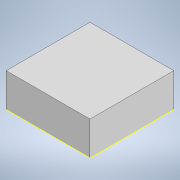
# Autodesk Inventor part: snapfit_lid_v02
Saved by Autodesk Inventor 2022 (Build 260153000, 153)
## iProperties
Created: 2022-03-20
Part Number: snapfit_lid_v02
Material: Generic
Document SubType Name: Modeling
Designer: LIMlab
Density: 1 g/cm^3
Appearance: Default
Author: LIMlab
Autodesk Inventor part; units mm, degrees
ref_plane "YZ Plane" through (0, 0, 0) normal (1, 0, 0) x (0, 1, 0)
ref_plane "XZ Plane" through (0, 0, 0) normal (0, 1, 0) x (-1, 0, 0)
ref_plane "XY Plane" through (0, 0, 0) normal (0, 0, 1) x (1, 0, 0)
sketch "Sketch1" plane through (0, 0, 0) normal (0, 1, 0) x (-1, 0, 0)
  line L0 (-2.5, 2.5) -> (2.5, 2.5)
  line L1 (2.5, 2.5) -> (2.5, -2.5)
  line L2 (2.5, -2.5) -> (-2.5, -2.5)
  line L3 (-2.5, -2.5) -> (-2.5, 2.5)
  line L4 (-2.5, 2.5) -> (2.5, -2.5) construction
  line L5 (2.5, 2.5) -> (-2.5, -2.5) construction
  point P0 (0, 0)
  dimension "d0" = 5
  dimension "d1" = 5
  constraints: 12 end point, 2 midpoint, 2 parallel, 1 horizontal, 1 perpendicular
  measures "d0" distance of L0.end L1.end
  measures "d1" distance of L1.end L2.end
extrude "Extrusion1" add sketch "Sketch1" along normal blind 10
shell "Shell1" thickness 1 removed faces 1 at (-0.8333, 10, -0.8333)
sketch "Sketch2" plane through (0, 10, 0) normal (0, 1, 0) x (1, 0, 0)
  line L0 (1.5, 1.5) -> (1.5, -1.5) projected
  line L1 (1.5, -1.5) -> (-1.5, -1.5) projected
  line L2 (-1.5, -1.5) -> (-1.5, 1.5) projected
  line L3 (-1.5, 1.5) -> (1.5, 1.5) projected
  line L4 (2.5, 2.5) -> (-2.5, 2.5) projected
  line L5 (-2.5, 2.5) -> (-2.5, -2.5) projected
  line L6 (-2.5, -2.5) -> (2.5, -2.5) projected
  line L7 (2.5, -2.5) -> (2.5, 2.5) projected
  line L8 (-2, 2) -> (-2, -2)
  line L9 (-2, -2) -> (2, -2)
  line L10 (2, -2) -> (2, 2)
  line L11 (2, 2) -> (-2, 2)
  point P0 (0, 0)
  dimension "d5" = 0.5
  constraints: 8 end point, 3 other
  measures "d5" distance between parallel lines of L2 L8
extrude "Extrusion2" add sketch "Sketch2" along normal blind 1 contours L11 L10 L9 L8
sketch "Sketch3" plane through (0, 10, 0) normal (0, 1, 0) x (1, 0, 0)
  line L0 (-2, -2) -> (-2, 2) projected
  line L1 (-2, 2) -> (2, 2) projected
  line L2 (2, 2) -> (2, -2) projected
  line L3 (2, -2) -> (-2, -2) projected
  line L4 (2.5, 2.5) -> (-2.5, 2.5) projected
  line L5 (-2.5, 2.5) -> (-2.5, -2.5) projected
  line L6 (-2.5, -2.5) -> (2.5, -2.5) projected
  line L7 (2.5, -2.5) -> (2.5, 2.5) projected
  line L8 (-1.5, -1.5) -> (-1.5, 1.5) projected
  line L9 (1.5, -1.5) -> (-1.5, -1.5) projected
  line L10 (1.5, 1.5) -> (1.5, -1.5) projected
  line L11 (-1.5, 1.5) -> (1.5, 1.5) projected
  point P0 (0, 0)
extrude "Extrusion3" cut sketch "Sketch3" along normal through all both and the other way through all contours L0 L1 L2 L3 | L7 L6 L5 L4 | L8 L11 L10 L9
extrude "Extrusion4" add sketch "Sketch3" along normal blind 1.5 contours L7 L6 L5 L4
sketch "Sketch4" plane through (0, 11.5, 0) normal (0, 1, 0) x (1, 0, 0)
  point P0 (0, 0)
sketch "Sketch5" plane through (0, 10, 0) normal (0, -1, 0) x (1, 0, 0)
  line L0 (-2, 2) -> (-2, -2) projected
  line L1 (-2, -2) -> (2, -2) projected
  line L2 (2, -2) -> (2, 2) projected
  line L3 (2, 2) -> (-2, 2) projected
  line L4 (-2.2, -2.2) -> (-2.2, 2.2)
  line L5 (-2.2, 2.2) -> (2.2, 2.2)
  line L6 (2.2, 2.2) -> (2.2, -2.2)
  line L7 (2.2, -2.2) -> (-2.2, -2.2)
  point P0 (0, 0)
  dimension "d12" = 0.2
  constraints: 8 end point, 3 other
  measures "d12" distance between parallel lines of L0 L4
extrude "Extrusion5" cut sketch "Sketch5" against normal blind 1.5 contours L3 L2 L1 L0 | L4 L5 L6 L7
sketch "Sketch6" plane through (0, 11.5, 0) normal (0, 1, 0) x (1, 0, 0)
  line L0 (-2.5, 2.5) -> (-2.5, -2.5) projected
  line L1 (-2.5, 2.5) -> (2.5, 2.5)
  line L2 (2.5, 2.5) -> (2.5, -2.5)
  line L3 (2.5, -2.5) -> (-2.5, -2.5)
  line L4 (-2.5, -2.5) -> (-2.5, 2.5)
  point P0 (0, 0)
  constraints: 8 end point, 2 parallel, 1 horizontal, 1 perpendicular
extrude "Extrusion6" add sketch "Sketch6" along normal blind 0.5
body "Solid1"
